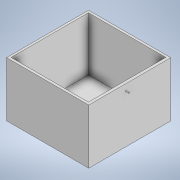
# Autodesk Inventor part: outerbox
Saved by Autodesk Inventor 2021 (Build 250183000, 183)
## iProperties
Created: 2023-06-07
Part Number: outerbox
Material: Generic
Document SubType Name: Modeling
Designer: badig
Density: 1 g/cm^3
Appearance: Default
Author: badig
Autodesk Inventor part; units mm, degrees
ref_plane "YZ Plane" through (0, 0, 0) normal (1, 0, 0) x (0, 1, 0)
ref_plane "XZ Plane" through (0, 0, 0) normal (0, 1, 0) x (-1, 0, 0)
ref_plane "XY Plane" through (0, 0, 0) normal (0, 0, 1) x (1, 0, 0)
sketch "Sketch1" plane through (0, 0, 0) normal (0, 0, 1) x (1, 0, 0)
  line L0 (-13.4502, 9.4461) -> (-471.2502, 9.4461)
  line L1 (-471.2502, 9.4461) -> (-471.2502, -295.3539)
  line L2 (-471.2502, -295.3539) -> (-13.4502, -295.3539)
  line L3 (-13.4502, -295.3539) -> (-13.4502, 9.4461)
  point P0 (0, 0)
  dimension "d0" = 457.8
  dimension "d1" = 304.8
  constraints: 8 end point, 2 parallel, 1 horizontal, 1 perpendicular
  measures "d0" distance of L2.end L1.end
  measures "d1" distance of L1.end L0.end
extrude "Extrusion1" add sketch "Sketch1" along normal blind 457
sketch "Sketch2" plane through (-471.2502, 9.4461, 0) normal (0, 1, 0) x (1, 0, 0)
  line L0 (12.104, -443.504) -> (442.7261, -443.504)
  line L1 (442.7261, -443.504) -> (442.7261, -12.8819)
  line L2 (442.7261, -12.8819) -> (12.104, -12.8819)
  line L3 (12.104, -12.8819) -> (12.104, -443.504)
  point P0 (471.2502, 0)
  constraints: 8 end point, 2 parallel, 1 horizontal, 1 perpendicular
extrude "Extrusion2" cut sketch "Sketch2" against normal blind 300
sketch "Sketch3" plane through (-13.4502, -295.3539, 0) normal (1, 0, 0) x (0, 0, -1)
  circle A0 centre (-248.4802, 267.8138) radius 4
  point P0 (0, 295.3539)
  dimension "d6" = 8
  constraints: 1 centre point
  measures "d6" diameter of A0
extrude "Extrusion3" add sketch "Sketch3" along normal blind 15
body "Solid1"
